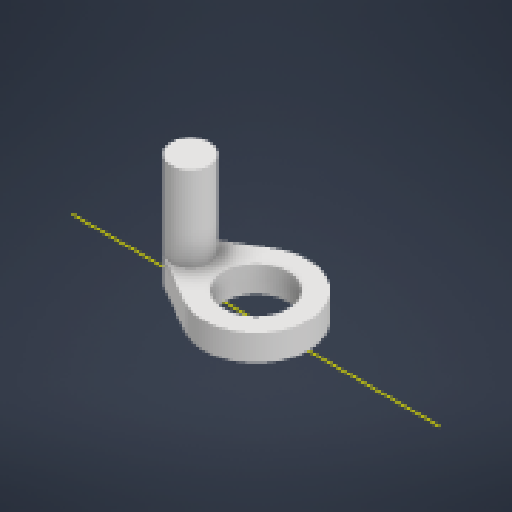
# Autodesk Inventor part: Рулевой толкатель на сервопривод
Saved by Autodesk Inventor 2026.2 (Build 302298000, 298)
## iProperties
Created: 2026-02-19
Part Number: Рулевой толкатель на сервопривод
Material: Типовые
Document SubType Name: Modeling
Designer: Leonid
Density: 1 g/cm^3
Appearance: По умолчанию
Author: Leonid
Autodesk Inventor part; units mm, degrees
ref_plane "YZ Plane" through (0, 0, 0) normal (1, 0, 0) x (0, 1, 0)
ref_plane "XZ Plane" through (0, 0, 0) normal (0, 1, 0) x (-1, 0, 0)
ref_plane "XY Plane" through (0, 0, 0) normal (0, 0, 1) x (1, 0, 0)
sketch "Эскиз1" plane through (0, 0, 0) normal (0, 1, 0) x (-1, 0, 0)
  circle A0 centre (0, 0) radius 2.45
  arc A1 (2, 3.4641) -> (2, -3.4641) centre (0, 0) ccw
  line L0 (5, 0) -> (5, 0) construction
  line L1 (5, 1.5) -> (5, 1.5)
  line L2 (5, -1.5) -> (5, -1.5)
  arc A2 (5, -1.5) -> (5, 1.5) centre (5, 0) ccw
  arc A3 (5, 1.5) -> (5, -1.5) centre (5, 0) ccw
  line L3 (8.6, 0) -> (-6.1, 0) projected
  line L4 (2, 3.4641) -> (5.75, 1.299)
  line L5 (2, -3.4641) -> (5.75, -1.299)
  arc A4 (5.75, -1.299) -> (5.75, 1.299) centre (5, 0) ccw
  point P0 (5, 0)
  point P1 (5, -1.5)
  dimension "d0" = 4.9
  dimension "d1" = 8
  dimension "d2" = 1.5
  dimension "d3" = 1.5
  dimension "d4" = 0
  dimension "d5" = 5
  constraints: 12 end point, 8 point on circle, 8 tangent, 5 centre point, 3 coincident, 1 collinear, 1 horizontal, 1 midpoint, 1 parallel
  measures "d0" diameter of A0
  measures "d1" diameter of A1
  measures "d2" radius of A2
  measures "d3" radius of A4
  measures "d4" distance of L0.end L0.start
  measures "d5" distance of point (0, 0) L0.end
extrude "Выдавливание1" add sketch "Эскиз1" along normal blind 2 contours L3 A3 A2 L5 A1 A0 | A0 L3 A1 L4 A2 A3
extrude "Выдавливание2" add sketch "Эскиз1" along normal blind 8.5 contours L3 A2 A3 | A3 A2 L3
sketch "Эскиз2" plane through (0, 0, 0) normal (0, 1, 0) x (-1, 0, 0)
  line L0 (14, 0) -> (-14, 0) projected
  point P0 (0, 0)
